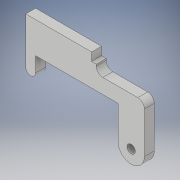
# Autodesk Inventor part: RackeSecondary
Saved by Autodesk Inventor 2019 (Build 230136000, 136)
## iProperties
Created: 2021-01-17
Part Number: RackeSecondary
Material: Типовые
Document SubType Name: Modeling
Designer: Dazer
Density: 1 g/cm^3
Appearance: По умолчанию
Author: Dazer
## iProperties of the stored document RackeSecondary_3DПЕЧАТЬ.ipt
Created: 2021-01-18
Part Number: RackeSecondary_3DПЕЧАТЬ
Material: Типовые
Document SubType Name: Modeling
Designer: Dazer
Density: 1 g/cm^3
Appearance: По умолчанию
Author: Dazer
Autodesk Inventor part; units mm, degrees
ref_plane "YZ Plane" through (0, 0, 0) normal (1, 0, 0) x (0, 1, 0)
ref_plane "XZ Plane" through (0, 0, 0) normal (0, 1, 0) x (-1, 0, 0)
ref_plane "XY Plane" through (0, 0, 0) normal (0, 0, 1) x (1, 0, 0)
sketch "Эскиз1" plane through (0, 0, 0) normal (0, 0, 1) x (1, 0, 0)
  line L0 (-20, 0) -> (0, 0)
  line L1 (-20, 0) -> (-20, 2.5)
  line L2 (-8.6117, 2.5) -> (-20, 2.5)
  spline S0 degree 3 poles (-5.9183, 5) (-5.9183, 4.7015) (-5.9968, 4.352) (-6.2503, 3.7878) (-6.4767, 3.4776) (-6.9505, 3.0315) (-7.2856, 2.8188) (-7.8976, 2.5753) (-8.2838, 2.5) (-8.6117, 2.5) knots 0 0 0 0 0.233745 0.233745 0.484283 0.484283 0.743265 0.743265 1 1 1 1
  line L3 (-5.9183, 2.5) -> (-5.9183, 5)
  line L4 (-5.9183, 2.5) -> (0, 2.5)
  line L5 (0, 0) -> (0, 2.5)
  line L6 (0, 0) -> (0, 2.5)
  line L7 (0, 2.5) -> (-20, 2.5)
  line L8 (-20, 0) -> (-20, 2.5)
  line L9 (0, 0) -> (1.4, 0)
  line L10 (1.4, 0) -> (1.4, -3.5)
  line L11 (-20, -13) -> (-17, -13)
  line L12 (-17, -7) -> (8, -7)
  line L13 (8, -13) -> (16, -13)
  line L14 (16, -3.5) -> (1.4, -3.5)
  line L15 (8, -13) -> (8, -17)
  line L16 (16, -17) -> (16, -13)
  arc A0 (8, -17) -> (16, -17) centre (12, -17) ccw
  circle A1 centre (12, -17) radius 1.25
  line L17 (16, -13) -> (16, -3.5)
  line L18 (8, -7) -> (8, -13)
  line L19 (-17, -7) -> (-17, -13)
  line L20 (-20, -13) -> (-20, 0)
  dimension "d7" = 2.5
  constraints: 30 end point, 4 vertical, 2 centre point, 2 collinear, 2 horizontal, 2 parallel, 2 point on circle, 1 coincident, 1 point on line
  measures "d7" diameter of A1
extrude "Выдавливание2" add sketch "Эскиз1" along normal blind 3 contours L1 L2 L7 L4 L5 L0 | L0 L9 L10 L14 L17 L13 L18 L12 L19 L11 L20 | L16 A0 L15 L13
sketch "Эскиз2" plane through (1.4, -3.5, 0) normal (0, 1, 0) x (1, 0, 0)
  line L0 (14.6, 0) -> (0, 0) projected
  line L1 (0, 0) -> (0, -3) projected
  line L2 (14.6, -3) -> (0, -3) projected
  line L3 (14.6, 0) -> (14.6, -3) projected
  point P0 (-1.4, 0)
extrude "Выдавливание3" add sketch "Эскиз2" along normal blind 1
fillet "Сопряжение3" radius 2 2 edges at (1.4, -2.5, 1.5) (16, -2.5, 1.5)
fillet "Сопряжение4" radius 1.5 2 edges at (-17, -13, 1.5) (-20, -13, 1.5)
